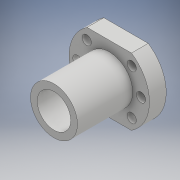
# Autodesk Inventor part: PowerScrewNut
Saved by Autodesk Inventor 2017 (Build 210142000, 142)
## iProperties
Created: 2017-03-12
Part Number: PowerScrewNut
Material: Generic
Document SubType Name: Modeling
Designer: umr
Density: 1 g/cm^3
Appearance: Default
Author: umr
Autodesk Inventor part; units mm, degrees
ref_plane "YZ Plane" through (0, 0, 0) normal (1, 0, 0) x (0, 1, 0)
ref_plane "XZ Plane" through (0, 0, 0) normal (0, 1, 0) x (-1, 0, 0)
ref_plane "XY Plane" through (0, 0, 0) normal (0, 0, 1) x (1, 0, 0)
sketch "Sketch1" plane through (0, 0, 0) normal (0, 1, 0) x (-1, 0, 0)
  circle A0 centre (0, 0) radius 14
  line L0 (13.2665, 20) -> (-13.2665, 20)
  line L1 (13.2665, -20) -> (-13.2665, -20)
  arc A1 (13.2665, -20) -> (13.2665, 20) centre (0, 0) ccw
  arc A2 (-13.2665, 20) -> (-13.2665, -20) centre (0, 0) ccw
  dimension "d1" = 28
  dimension "d2" = 20
  dimension "d3" = 20
  dimension "d19" = 24
  constraints: 4 end point, 4 point on circle, 3 centre point, 2 coincident, 2 horizontal
  measures "d1" diameter of A0
  measures "d2" distance from line of point (0, 0) L0
  measures "d3" distance from line of point (0, 0) L1
  measures "d19" radius of A1
extrude "Extrusion1" add sketch "Sketch1" along normal blind 10
sketch "Sketch2" plane through (0, 10, 0) normal (0, 1, 0) x (1, 0, 0)
  circle A0 centre (0, 0) radius 14 projected
  line L0 (-13.2665, -20) -> (13.2665, -20) projected
  arc A1 (13.2665, -20) -> (13.2665, 20) centre (0, 0) ccw projected
  line L1 (13.2665, 20) -> (-13.2665, 20) projected
  arc A2 (-13.2665, 20) -> (-13.2665, -20) centre (0, 0) ccw projected
  circle A3 centre (-19, 0) radius 2.75
  circle A4 centre (-13.435, 13.435) radius 2.75
  circle A5 centre (-13.435, -13.435) radius 2.75
  line L2 (0, -20) -> (0, 20)
  line L3 (13.2665, 20) -> (-13.2665, 20) projected
  circle A6 centre (19, 0) radius 2.75
  circle A7 centre (13.435, 13.435) radius 2.75
  circle A8 centre (13.435, -13.435) radius 2.75
  dimension "d6" = 5.5
  dimension "d7" = 0
  dimension "d8" = 24
  dimension "d9" = 28
  dimension "d10" = 19
  dimension "d11" = 5.5
  dimension "d12" = 13.435
  dimension "d13" = 13.435
  dimension "d14" = 5.5
  dimension "d15" = 13.435
  dimension "d16" = 13.435
  dimension "d20" = 38
  constraints: 6 centre point, 3 symmetric about line, 2 end point, 2 midpoint, 3 other
  measures "d6" diameter of A3
  measures "d7" vertical distance of A3.centre point (0, 0)
  measures "d8" radius of A2
  measures "d9" diameter of A0
  measures "d10" distance of point (0, 0) A3.centre
  measures "d11" diameter of A4
  measures "d12" horizontal distance of point (0, 0) A4.centre
  measures "d13" horizontal distance of point (0, 0) A4.centre
  measures "d14" diameter of A5
  measures "d15" horizontal distance of point (0, 0) A5.centre
  measures "d16" horizontal distance of point (0, 0) A5.centre
  measures "d20" distance of A6.centre A3.centre
extrude "Extrusion2" cut sketch "Sketch2" against normal blind 10 contours A3 | A4 | A5 | A6 | A7 | A8
sketch "Sketch3" plane through (0, 10, 0) normal (0, 1, 0) x (1, 0, 0)
  circle A0 centre (0, 0) radius 14 projected
  circle A1 centre (0, 0) radius 10
  dimension "d21" = 20
  constraints: 1 centre point, 1 coincident
  measures "d21" diameter of A1
extrude "Extrusion3" add sketch "Sketch3" against normal blind 43
equation "\"d10\" = 0.25 * d9 + 0.5 * d8"
equation "\"d12\" = 0.707107 * d10"
equation "\"d13\" = d12"
equation "\"d15\" = d13"
equation "\"d16\" = d12"
body "Solid1"
